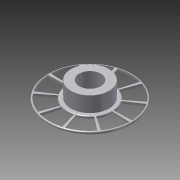
# Autodesk Inventor part: Spool Half
Saved by Autodesk Inventor 2015 (Build 190159000, 159)
## iProperties
Created: 2015-10-04
Part Number: Spool Half
Material: ABS Plastic
Document SubType Name: Modeling
Designer: Kurtis
Density: 1.06 g/cm^3
Appearance: Smooth - White
Mass: 119.257 g
Surface Area: 817.934 cm^2
Volume: 112.507 cm^3
Author: Kurtis
Autodesk Inventor part; units mm, degrees
ref_plane "YZ Plane" through (0, 0, 0) normal (1, 0, 0) x (0, 1, 0)
ref_plane "XZ Plane" through (0, 0, 0) normal (0, 1, 0) x (-1, 0, 0)
ref_plane "XY Plane" through (0, 0, 0) normal (0, 0, 1) x (1, 0, 0)
sketch "Sketch1" plane through (0, 0, 0) normal (0, 0, 1) x (1, 0, 0)
  circle A0 centre (0, 0) radius 100
  circle A1 centre (0, 0) radius 42.25
  dimension "d0" = 200
  dimension "d1" = 84.5
  constraints: 2 centre point, 2 coincident
  measures "d0" diameter of A0
  measures "d1" diameter of A1
extrude "Main Body" add sketch "Sketch1" along normal blind 5
sketch "Sketch2" plane through (0, 0, 5) normal (0, 0, 1) x (1, 0, 0)
  circle A0 centre (0, 0) radius 45.25
  circle A1 centre (0, 0) radius 42.25
  dimension "d4" = 90.5
  dimension "d10" = 84.5
  constraints: 2 centre point, 2 coincident
  measures "d4" diameter of A0
  measures "d10" diameter of A1
extrude "Indent (Deprecateds)" add sketch "Sketch2" along normal blind 16
sketch "Sketch3" plane through (0, 0, 21) normal (0, 0, 1) x (1, 0, 0)
  circle A0 centre (0, 0) radius 25.875
  circle A1 centre (0, 0) radius 45.25
  dimension "d7" = 51.75
  dimension "d11" = 90.5
  constraints: 2 centre point, 2 coincident
  measures "d7" diameter of A0
  measures "d11" diameter of A1
extrude "Hub/Connector" add sketch "Sketch3" along normal blind 20.5 and the other way blind 21
sketch "Sketch5" plane through (0, 0, 5) normal (0, 0, 1) x (1, 0, 0)
  circle A0 centre (0, 0) radius 100 construction
  line L0 (0, 100) -> (0, 45.25) construction
  circle A1 centre (0, 0) radius 45.25 construction
  line L1 (0, 72.625) -> (0, 100) construction
  line L2 (0, 86.3125) -> (0, 100) construction
  line L3 (0, 93.1562) -> (-36.3581, 93.1562) construction
  line L4 (0, 93.1562) -> (36.3581, 93.1562) construction
  line L5 (0, 72.625) -> (0, 45.25) construction
  line L6 (0, 58.9375) -> (0, 45.25) construction
  line L7 (0, 52.0938) -> (85.3595, 52.0938) construction
  line L8 (0, 52.0938) -> (-85.3595, 52.0938) construction
  circle A2 centre (0, 0) radius 97 construction
  arc A3 (27.0354, 93.1562) -> (-27.0354, 93.1562) centre (0, 0) ccw
  line L9 (27.0354, 93.1562) -> (0, 0) construction
  line L10 (0, 0) -> (-27.0354, 93.1562) construction
  arc A4 (15.1184, 52.0938) -> (-15.1184, 52.0938) centre (0, 0) ccw
  line L11 (-27.0354, 93.1562) -> (-15.1184, 52.0938)
  line L12 (15.1184, 52.0938) -> (27.0354, 93.1562)
  arc A5 (-32.8838, 91.256) -> (-76.628, 59.474) centre (0, 0) ccw
  arc A6 (-18.3889, 51.0311) -> (-42.851, 33.2583) centre (0, 0) ccw
  line L13 (-76.628, 59.474) -> (-42.851, 33.2583)
  line L14 (-18.3889, 51.0311) -> (-32.8838, 91.256)
  arc A7 (-80.2425, 54.4991) -> (-96.9513, 3.0747) centre (0, 0) ccw
  arc A8 (-44.8723, 30.4763) -> (-54.216, 1.7194) centre (0, 0) ccw
  line L15 (-96.9513, 3.0747) -> (-54.216, 1.7194)
  line L16 (-44.8723, 30.4763) -> (-80.2425, 54.4991)
  arc A9 (-96.9513, -3.0747) -> (-80.2425, -54.4991) centre (0, 0) ccw
  arc A10 (-54.216, -1.7194) -> (-44.8723, -30.4763) centre (0, 0) ccw
  line L17 (-80.2425, -54.4991) -> (-44.8723, -30.4763)
  line L18 (-54.216, -1.7194) -> (-96.9513, -3.0747)
  arc A11 (-76.628, -59.474) -> (-32.8838, -91.256) centre (0, 0) ccw
  arc A12 (-42.851, -33.2583) -> (-18.3889, -51.0311) centre (0, 0) ccw
  line L19 (-32.8838, -91.256) -> (-18.3889, -51.0311)
  line L20 (-42.851, -33.2583) -> (-76.628, -59.474)
  arc A13 (-27.0354, -93.1562) -> (27.0354, -93.1562) centre (0, 0) ccw
  arc A14 (-15.1184, -52.0938) -> (15.1184, -52.0938) centre (0, 0) ccw
  line L21 (27.0354, -93.1562) -> (15.1184, -52.0938)
  line L22 (-15.1184, -52.0938) -> (-27.0354, -93.1562)
  arc A15 (32.8838, -91.256) -> (76.628, -59.474) centre (0, 0) ccw
  arc A16 (18.3889, -51.0311) -> (42.851, -33.2583) centre (0, 0) ccw
  line L23 (76.628, -59.474) -> (42.851, -33.2583)
  line L24 (18.3889, -51.0311) -> (32.8838, -91.256)
  arc A17 (80.2425, -54.4991) -> (96.9513, -3.0747) centre (0, 0) ccw
  arc A18 (44.8723, -30.4763) -> (54.216, -1.7194) centre (0, 0) ccw
  line L25 (96.9513, -3.0747) -> (54.216, -1.7194)
  line L26 (44.8723, -30.4763) -> (80.2425, -54.4991)
  arc A19 (96.9513, 3.0747) -> (80.2425, 54.4991) centre (0, 0) ccw
  arc A20 (54.216, 1.7194) -> (44.8723, 30.4763) centre (0, 0) ccw
  line L27 (80.2425, 54.4991) -> (44.8723, 30.4763)
  line L28 (54.216, 1.7194) -> (96.9513, 3.0747)
  arc A21 (76.628, 59.474) -> (32.8838, 91.256) centre (0, 0) ccw
  arc A22 (42.851, 33.2583) -> (18.3889, 51.0311) centre (0, 0) ccw
  line L29 (32.8838, 91.256) -> (18.3889, 51.0311)
  line L30 (42.851, 33.2583) -> (76.628, 59.474)
  dimension "d34" = 194
  dimension "d36" = 41.0625
  dimension "d37" = 54.2432
  dimension "d40" = 360
  constraints: 62 end point, 45 point on circle, 20 centre point, 12 coincident, 6 collinear, 5 midpoint, 5 point on line, 2 perpendicular, 1 vertical, 1 vertical alignment, 105 other
  measures "d36" vertical distance of L12.start L9.start
  measures "d37" radius of A4
extrude "Cheap Hole Pattern" cut sketch "Sketch5" against normal blind 68
sketch "Sketch7" plane through (0, 0, 0) normal (0, 0, -1) x (-1, 0, 0)
  circle A0 centre (0, 0) radius 25.875 construction
  line L0 (0, -25.875) -> (0, -28.375) construction
  line L1 (0, -28.375) -> (5, -28.375) construction
  line L2 (5, -28.375) -> (-5, -28.375)
  line L3 (0, -28.375) -> (0, -41.375) construction
  line L4 (0, -41.375) -> (7.5, -41.375) construction
  line L5 (7.5, -41.375) -> (-7.5, -41.375)
  line L6 (-7.5, -41.375) -> (-5, -28.375)
  line L7 (5, -28.375) -> (7.5, -41.375)
  line L8 (16.1089, -23.8882) -> (23.6803, -34.7474)
  line L9 (23.6803, -34.7474) -> (9.9771, -40.8485)
  line L10 (9.9771, -40.8485) -> (6.9734, -27.9555)
  line L11 (16.1089, -23.8882) -> (6.9734, -27.9555)
  line L12 (24.4324, -15.2709) -> (35.7661, -22.1117)
  line L13 (35.7661, -22.1117) -> (25.7291, -33.2589)
  line L14 (25.7291, -33.2589) -> (17.7411, -22.7023)
  line L15 (24.4324, -15.2709) -> (17.7411, -22.7023)
  line L16 (28.5313, -4.0131) -> (41.6676, -5.6527)
  line L17 (41.6676, -5.6527) -> (37.0323, -19.9185)
  line L18 (37.0323, -19.9185) -> (25.4411, -13.5236)
  line L19 (28.5313, -4.0131) -> (25.4411, -13.5236)
  line L20 (27.6969, 7.9386) -> (40.3644, 11.7838)
  line L21 (40.3644, 11.7838) -> (41.9323, -3.134)
  line L22 (41.9323, -3.134) -> (28.7422, -2.0066)
  line L23 (27.6969, 7.9386) -> (28.7422, -2.0066)
  line L24 (22.0735, 18.5176) -> (32.0818, 27.1827)
  line L25 (32.0818, 27.1827) -> (39.5818, 14.1923)
  line L26 (39.5818, 14.1923) -> (27.0735, 9.8574)
  line L27 (22.0735, 18.5176) -> (27.0735, 9.8574)
  line L28 (12.6333, 25.8948) -> (18.252, 37.8815)
  line L29 (18.252, 37.8815) -> (30.3872, 29.0647)
  line L30 (30.3872, 29.0647) -> (20.7235, 20.0169)
  line L31 (12.6333, 25.8948) -> (20.7235, 20.0169)
  line L32 (1.0088, 28.7945) -> (1.2662, 42.0302)
  line L33 (1.2662, 42.0302) -> (15.9385, 38.9115)
  line L34 (15.9385, 38.9115) -> (10.7902, 26.7154)
  line L35 (1.0088, 28.7945) -> (10.7902, 26.7154)
  line L36 (-10.7902, 26.7154) -> (-15.9385, 38.9115)
  line L37 (-15.9385, 38.9115) -> (-1.2662, 42.0302)
  line L38 (-1.2662, 42.0302) -> (-1.0088, 28.7945)
  line L39 (-10.7902, 26.7154) -> (-1.0088, 28.7945)
  line L40 (-20.7235, 20.0169) -> (-30.3872, 29.0647)
  line L41 (-30.3872, 29.0647) -> (-18.252, 37.8815)
  line L42 (-18.252, 37.8815) -> (-12.6333, 25.8948)
  line L43 (-20.7235, 20.0169) -> (-12.6333, 25.8948)
  line L44 (-27.0735, 9.8574) -> (-39.5818, 14.1923)
  line L45 (-39.5818, 14.1923) -> (-32.0818, 27.1827)
  line L46 (-32.0818, 27.1827) -> (-22.0735, 18.5176)
  line L47 (-27.0735, 9.8574) -> (-22.0735, 18.5176)
  line L48 (-28.7422, -2.0066) -> (-41.9323, -3.134)
  line L49 (-41.9323, -3.134) -> (-40.3644, 11.7838)
  line L50 (-40.3644, 11.7838) -> (-27.6969, 7.9386)
  line L51 (-28.7422, -2.0066) -> (-27.6969, 7.9386)
  line L52 (-25.4411, -13.5236) -> (-37.0323, -19.9185)
  line L53 (-37.0323, -19.9185) -> (-41.6676, -5.6527)
  line L54 (-41.6676, -5.6527) -> (-28.5313, -4.0131)
  line L55 (-25.4411, -13.5236) -> (-28.5313, -4.0131)
  line L56 (-17.7411, -22.7023) -> (-25.7291, -33.2589)
  line L57 (-25.7291, -33.2589) -> (-35.7661, -22.1117)
  line L58 (-35.7661, -22.1117) -> (-24.4324, -15.2709)
  line L59 (-17.7411, -22.7023) -> (-24.4324, -15.2709)
  line L60 (-6.9734, -27.9555) -> (-9.9771, -40.8485)
  line L61 (-9.9771, -40.8485) -> (-23.6803, -34.7474)
  line L62 (-23.6803, -34.7474) -> (-16.1089, -23.8882)
  line L63 (-6.9734, -27.9555) -> (-16.1089, -23.8882)
  dimension "d48" = 2.5
  dimension "d49" = 5
  dimension "d50" = 10
  dimension "d51" = 13
  dimension "d52" = 7.5
  dimension "d53" = 15
  dimension "d54" = 360
  dimension "d55" = 41.375
  constraints: 128 end point, 3 perpendicular, 2 point on line, 1 vertical, 1 vertical alignment, 123 other
  measures "d48" distance of L0.start L0.end
  measures "d49" distance of L0.end L1.end
  measures "d50" distance of L1.end L2.end
  measures "d51" distance of L0.end L3.end
  measures "d52" distance of L3.end L4.end
  measures "d53" distance of L4.end L5.end
  measures "d55" distance from line of point (0, 0) L21
extrude "InnerSpool" cut sketch "Sketch7" against normal blind 25
fillet "Outer Fillet" radius 2 1 edges at (-100, 0, 5)
fillet "Inner Fillet" radius 2 10 edges at (31.8834, -43.8837, 5) (51.5884, -16.7621, 5) (51.5884, 16.7621, 5) (31.8834, 43.8837, 5) (0, 54.2432, 5) (-31.8834, 43.8837, 5) (-51.5884, 16.7621, 5) (-51.5884, -16.7621, 5) (0, -54.2432, 5) (-31.8834, -43.8837, 5)
sketch "Sketch9" plane through (-7.5, -41.375, 0) normal (0, 1, 0) x (1, 0, 0)
  line L0 (12.5, 0) -> (12.5, -25) projected
  circle A0 centre (12.5, -6.6129) radius 1
  point P0 (7.5, 0)
  dimension "d65" = 2
  constraints: 1 centre point, 1 point on line
  measures "d65" diameter of A0
extrude "Filament Hole" cut sketch "Sketch9" along normal mid plane 14
body "Solid1"
